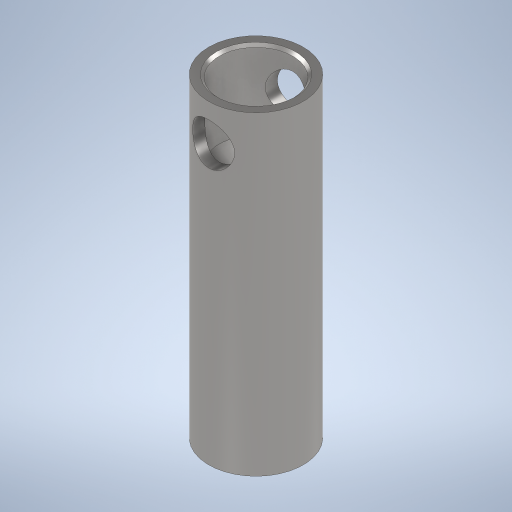
# Autodesk Inventor part: RS-STT-103
Saved by Autodesk Inventor 2024 (Build 280153000, 153)
## iProperties
Created: 2024-05-23
Part Number: RS-STT-103
Material: 11 110 (1.0721)
Document SubType Name: Modeling
Designer: Roman Suk
Density: 7.85 g/cm^3
Appearance: Semi-Polished
Mass: 87.1358 g
Surface Area: 51.3151 cm^2
Volume: 11.1001 cm^3
Description: Matice s posuvnou rukojetí
MASSSFP: 123,82 g
SFP: KR 18h11-65 ČSN 42 6510
Author: Roman Suk
Autodesk Inventor part; units mm, degrees
ref_plane "YZ Plane" through (0, 0, 0) normal (1, 0, 0) x (0, 1, 0)
ref_plane "XZ Plane" through (0, 0, 0) normal (0, 1, 0) x (-1, 0, 0)
ref_plane "XY Plane" through (0, 0, 0) normal (0, 0, 1) x (1, 0, 0)
sketch "Sketch2" plane through (0, 0, 0) normal (0, 1, 0) x (-1, 0, 0)
  circle A0 centre (0, 0) radius 9
  dimension "d2" = 18
  constraints: 2 coincident, 1 centre point
  measures "d2" diameter of A0
extrude "Extrusion2" add sketch "Sketch2" along normal blind 60
hole "Hole1" at (0, 0, 0) direction (0, 1, 0) diameter 8.376 depth 25 tip angle 118 countersink diameter 10 countersink angle 118 thread size "M10x1.5" class "6H" standard "ISO Metric profile"
sketch "Sketch3" plane through (0, 60, 0) normal (0, 1, 0) x (1, 0, 0)
  point P0 (0, 0)
  point P1 (0, 0)
  constraints: 1 coincident
hole "Hole2" at (0, 60, 0) direction (0, -1, 0) diameter 14 depth 15 tip angle 118
sketch "Sketch4" plane through (0, 0, 0) normal (0, 0, 1) x (1, 0, 0)
  circle A0 centre (0, 53) radius 4
  line L0 (9, 60) -> (-9, 60) projected
  point P0 (0, 0)
  point P1 (0, 60)
  dimension "d20" = 8
  dimension "d21" = 7
  constraints: 1 centre point, 1 midpoint, 1 vertical alignment
  measures "d20" diameter of A0
  measures "d21" distance from line of L0 A0.centre
extrude "Extrusion3" cut sketch "Sketch4" along normal through all both and the other way through all
chamfer "Chamfer3" distance 0.5 angle 45 1 edges at (0, 60, -7)
sketch "Sketch6" plane through (0, 60, 0) normal (0, 1, 0) x (1, 0, 0)
  circle A0 centre (0, 0) radius 9 projected
  line L0 (-9, 0) -> (9, 0)
  line L1 (9, 0) -> (9, 9)
  line L2 (9, 9) -> (-9, 9)
  line L3 (-9, 9) -> (-9, 0)
  dimension "d38" = 9
  dimension "d39" = 18
  constraints: 8 end point, 2 parallel, 2 point on circle, 1 horizontal, 1 perpendicular
  measures "d38" distance of L2.end L0.start
  measures "d39" distance of L1.end L2.end
extrude "Extrusion5" [suppressed]
body "Solid2"
